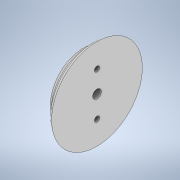
# Autodesk Inventor part: gearboxmotorconnection
Saved by Autodesk Inventor 2022 (Build 260153000, 153)
## iProperties
Created: 2021-08-23
Part Number: gearboxmotorconnection
Material: Generic
Document SubType Name: Modeling
Designer: Ferdinand Hubbard
Density: 1 g/cm^3
Appearance: Default
Author: Ferdinand Hubbard
Autodesk Inventor part; units mm, degrees
ref_plane "YZ Plane" through (0, 0, 0) normal (1, 0, 0) x (0, 1, 0)
ref_plane "XZ Plane" through (0, 0, 0) normal (0, 1, 0) x (-1, 0, 0)
ref_plane "XY Plane" through (0, 0, 0) normal (0, 0, 1) x (1, 0, 0)
sketch "Sketch1" plane through (0, 0, 0) normal (0, 1, 0) x (-1, 0, 0)
  line L0 (0, 0) -> (0, -18) construction
  line L1 (0, 0) -> (-8, 0)
  line L2 (-8, 0) -> (-8, -27) construction
  line L3 (-2.3867, -20.6851) -> (-5.6133, -24.3149)
  arc A0 (0, -18.852) -> (-2.3867, -20.6851) centre (3.5925, -26) ccw
  arc A1 (-8, -26.148) -> (-5.6133, -24.3149) centre (-11.5925, -19) ccw
  line L4 (0, 0) -> (0, -18.852)
  line L5 (-8, 0) -> (-8, -26.148)
  dimension "d0" = 18
  dimension "d1" = 8
  dimension "d2" = 27
  dimension "d3" = 8
  constraints: 12 end point, 4 point on circle, 4 point on line, 2 centre point, 2 collinear, 2 tangent, 2 vertical, 1 equal radius, 1 horizontal
  measures "d0" distance of L0.start L0.end
  measures "d1" distance of L0.start L1.end
  measures "d2" distance of L1.end L2.end
  measures "d3" radius of A0
revolve "Revolution1" add sketch "Sketch1" angle 360 about axis through (0, 0, 0) along (1, 0, 0)
sketch "Sketch2" plane through (0, 0, 0) normal (-1, 0, 0) x (0, 0, 1)
  circle A0 centre (0, 0) radius 2.5
  line L0 (0, 0) -> (0, 12.5) construction
  circle A1 centre (0, 12.5) radius 1.5
  line L1 (0, 0) -> (0, -12.5) construction
  circle A2 centre (0, -12.5) radius 1.5
  dimension "d5" = 5
  dimension "d6" = 12.5
  dimension "d7" = 12.5
  dimension "d8" = 3
  dimension "d9" = 3
  constraints: 4 end point, 3 centre point, 3 coincident, 2 vertical
  measures "d5" diameter of A0
  measures "d6" distance of L0.start L0.end
  measures "d7" distance of L0.start L1.end
  measures "d8" diameter of A1
  measures "d9" diameter of A2
extrude "Extrusion1" cut sketch "Sketch2" against normal blind 10
body "Solid1"
